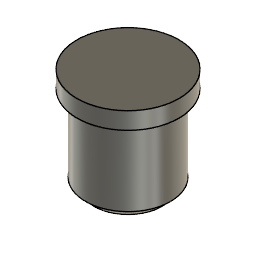
Peg Connection v2 (Autodesk Fusion 360 design; units mm, degrees)
part number: 2026-01-19-14-38-02-559
Autodesk Fusion 360 part; units mm, degrees
sketch "Sketch4" plane through (0, 0, 0) normal (0, 0, 1) x (1, 0, 0)
  circle A0 centre (0, 0) radius 12.7
  dimension "d28" = 25.4
  constraint coincident A0.centre origin
  measures "d28" diameter of A0
extrude "Extrude4" add sketch "Sketch4" along normal blind 25.4
sketch "Sketch5" plane through (0, 0, 25.4) normal (0, 0, 1) x (-1, 0, 0)
  circle A0 centre (0, 0) radius 12.7
  circle A1 centre (0, 0) radius 15.24
  constraint concentric A0 A1
extrude "Extrude5" add sketch "Sketch5" along normal blind 5.08 contours A0 | A1
chamfer "Chamfer2" distance 2.54 angle 45 1 edges at (-11.8406, -4.5925, 0)
